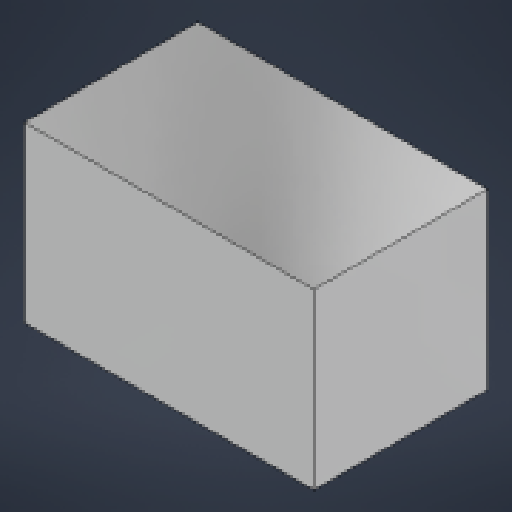
# Autodesk Inventor part: PLATE,NUTBLOCK,BACK
Saved by Autodesk Inventor 2026.1 (Build 301233020, 233B)
## iProperties
Created: 2026-01-29
Part Number: PLATE,NUTBLOCK,BACK
Material: Aluminum 6061
Document SubType Name: Sheet Metal
Designer: Owen L
Density: 2.7 g/cm^3
Sheet Metal Rule: Default
Appearance: Aluminum - Flat
Author: Owen L
Autodesk Inventor part; units mm, degrees
ref_plane "YZ Plane" through (0, 0, 0) normal (1, 0, 0) x (0, 1, 0)
ref_plane "XZ Plane" through (0, 0, 0) normal (0, 1, 0) x (-1, 0, 0)
ref_plane "XY Plane" through (0, 0, 0) normal (0, 0, 1) x (1, 0, 0)
sketch "Sketch1" plane through (0, 0, 0) normal (0, 1, 0) x (-1, 0, 0)
  line L0 (-9.525, 4.7625) -> (9.525, 4.7625)
  line L1 (9.525, 4.7625) -> (9.525, -4.7625)
  line L2 (9.525, -4.7625) -> (-9.525, -4.7625)
  line L3 (-9.525, -4.7625) -> (-9.525, 4.7625)
  line L4 (-9.525, 4.7625) -> (9.525, -4.7625) construction
  line L5 (9.525, 4.7625) -> (-9.525, -4.7625) construction
  point P0 (0, 0)
  dimension "d0" = 19.05
  dimension "d1" = 9.525
  measures "d0" distance of L1.end L2.end
  measures "d1" distance of L0.end L1.end
extrude "Plate1" add sketch "Sketch1" along normal blind 9.525
sketch "Sketch2" plane through (9.525, 0, -4.7625) normal (0, 0, -1) x (-1, 0, 0)
  line L0 (0, 0) -> (19.05, 0) construction
  line L1 (9.525, 0) -> (9.525, 9.525) construction
  line L2 (19.05, 9.525) -> (0, 9.525) construction
  point P0 (3.175, 6.35)
  point P1 (15.875, 6.35)
  dimension "d3" = 12.7
  dimension "d4" = 6.35
  constraints: 2 end point, 1 horizontal alignment, 1 midpoint, 1 symmetric about line
  measures "d3" distance of point (15.875, 6.35) point (3.175, 6.35)
  measures "d4" distance from line of L0 point (3.175, 6.35)
hole "Hole1" at (6.35, 6.35, -4.7625) at (-6.35, 6.35, -4.7625) direction (0, 0, 1) diameter 3.9624 end through all thread size "10-32 UNF" class "2B" standard "ANSI Unified Screw Threads"
sketch "Sketch3" plane through (0, 9.525, 0) normal (0, 1, 0) x (1, 0, 0)
  line L0 (-9.525, 4.7625) -> (9.525, 4.7625) projected
  point P0 (0, 0)
  point P1 (0, -1.5875)
  dimension "d19" = 6.35
  constraints: 1 vertical alignment
  measures "d19" distance from line of L0 point (0, -1.588)
hole "Hole2" at (0, 9.525, 1.5875) direction (0, -1, 0) diameter 3.9624 end through all thread size "10-32 UNF" class "2B" standard "ANSI Unified Screw Threads"
fillet "Corner Round1" radius 1.5875 4 edges at (-9.525, 4.7625, -4.7625) (-9.525, 4.7625, 4.7625) (9.525, 4.7625, -4.7625) (9.525, 4.7625, 4.7625)
equation "\"d10\" = Thickness"
equation "\"d2\" = Thickness"
equation "\"BendRadius\" = Thickness"
equation "\"BendReliefWidth\" = Thickness"
equation "\"BendReliefDepth\" = 0.5 * Thickness"
equation "\"CornerReliefSize\" = 4 * Thickness"
equation "\"MinimumRemnant\" = 2 * Thickness"
equation "\"TransitionRadius\" = BendRadius"
equation "\"JacobiRadiusSize\" = BendRadius"
equation "\"GapSize\" = Thickness"
equation "\"Thickness\" = 9.525"
body "Solid1"
